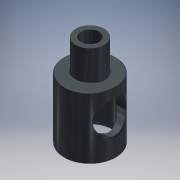
# Autodesk Inventor part: Component 26 (Valve Cup)
Saved by Autodesk Inventor 2018 (Build 220112000, 112)
## iProperties
Created: 2023-03-25
Part Number: Component 26 (Valve Cup)
Material: Generic
Document SubType Name: Modeling
Designer: Habib Mohamed
Density: 1 g/cm^3
Appearance: Iron Gray
Author: Habib Mohamed
Autodesk Inventor part; units mm, degrees
ref_plane "YZ Plane" through (0, 0, 0) normal (1, 0, 0) x (0, 1, 0)
ref_plane "XZ Plane" through (0, 0, 0) normal (0, 1, 0) x (-1, 0, 0)
ref_plane "XY Plane" through (0, 0, 0) normal (0, 0, 1) x (1, 0, 0)
sketch "Sketch1" plane through (0, 0, 0) normal (1, 0, 0) x (0, 1, 0)
  line L0 (19.45, 1.9) -> (11.05, 1.9)
  line L1 (11.05, 1.9) -> (11.05, 3.8)
  line L2 (10.85, 4) -> (1.2699, 4)
  line L3 (0.9164, 4.1464) -> (0.3614, 4.7014)
  line L4 (0.22, 4.76) -> (0.2, 4.76)
  line L5 (0, 4.76) -> (0, 5.5) construction
  line L6 (0.2, 5.5) -> (12.85, 5.5)
  line L7 (13.05, 5.3) -> (13.05, 3.2)
  line L8 (13.25, 3) -> (19.45, 3)
  line L9 (19.45, 3) -> (19.45, 1.9)
  line L10 (0, 0) -> (36.4662, 0) construction
  line L11 (0, 4.96) -> (0, 5.3) construction
  arc A0 (0.2, 5.5) -> (0, 5.3) centre (0.2, 5.3) ccw
  arc A1 (0, 4.96) -> (0.2, 4.76) centre (0.2, 4.96) ccw
  arc A2 (0.3614, 4.7014) -> (0.22, 4.76) centre (0.22, 4.56) ccw
  arc A3 (0.9164, 4.1464) -> (1.2699, 4) centre (1.2699, 4.5) ccw
  line L12 (0, 5.3) -> (0, 4.96)
  arc A4 (13.05, 3.2) -> (13.25, 3) centre (13.25, 3.2) ccw
  arc A5 (13.05, 5.3) -> (12.85, 5.5) centre (12.85, 5.3) ccw
  arc A6 (11.05, 3.8) -> (10.85, 4) centre (10.85, 3.8) ccw
  point P0 (11.05, 4)
  point P1 (13.05, 5.5)
  point P2 (13.05, 3)
  dimension "d0" = 13.05
  dimension "d1" = 6.4
  dimension "d2" = 11.05
  dimension "d3" = 45
  dimension "d4" = 0.74
  dimension "d5" = 1.9
  dimension "d6" = 3
  dimension "d7" = 4
  dimension "d8" = 5.5
  dimension "d9" = 0.2
  dimension "d10" = 0.2
  dimension "d11" = 0.5
  dimension "d12" = 0.22
  dimension "d21" = 0.2
  constraints: 26 end point, 15 point on circle, 14 tangent, 10 point on line, 7 centre point, 7 perpendicular, 3 equal radius, 2 horizontal, 1 collinear, 1 parallel, 1 vertical
  measures "d0" distance of L5.end point (13.05, 5.5)
  measures "d1" distance of point (13.05, 3) L8.end
  measures "d2" distance between parallel lines of L1 L5
  measures "d3" angle of L3 L5
  measures "d4" distance between parallel lines of L6 L4
  measures "d5" distance between parallel lines of L0 L10
  measures "d6" distance between parallel lines of L8 L10
  measures "d7" distance between parallel lines of L10 L2
  measures "d8" distance between parallel lines of L10 L6
  measures "d9" radius of A0
  measures "d10" radius of A2
  measures "d11" radius of A3
  measures "d12" distance from line of A2.centre L11
  measures "d21" radius of A4
revolve "Revolution1" add sketch "Sketch1" angle 360 about axis through (0, 0, 0) along (0, 1, 0)
sketch "Sketch2" plane through (0, 0, 0) normal (1, 0, 0) x (0, 1, 0)
  circle A0 centre (7.55, 0) radius 3.5
  point P0 (0, 0)
  dimension "d14" = 7
  dimension "d15" = 7.55
  constraints: 1 centre point
  measures "d14" diameter of A0
  measures "d15" distance of point (0, 0) A0.centre
extrude "Extrusion1" cut sketch "Sketch2" along normal blind 10
chamfer "Chamfer1" distance 0.2 angle 45 1 edges at (5.5, 4.05, -0.006)
body "Solid1"
